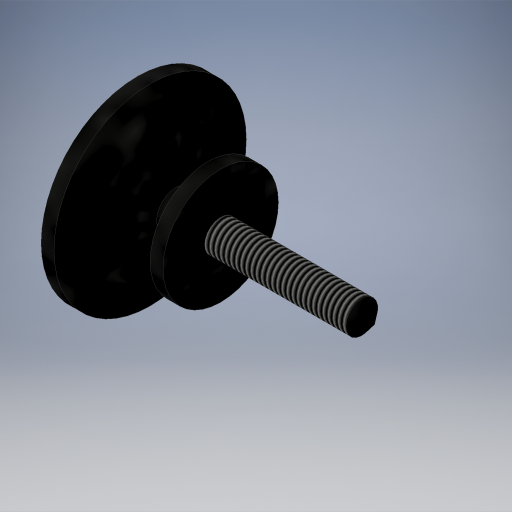
# Autodesk Inventor part: BT002_trajan20_22
Saved by Autodesk Inventor 2023 (Build 270158000, 158)
## iProperties
Company: HTBLA Kaindorf
RuleStatus: InUse
Created: 2022-11-02
Part Number: BT002_trajan20_22
Project: Zeichenmaschine_neu
Material: Kunststoff, undurchsichtig Schwarz
Description: Fuß
Document SubType Name: Modeling
Designer: trajan20
Density: 0.952 g/cm^3
Appearance: Glatt - Schwarz
Mass: 3.50123 g
Surface Area: 26.4974 cm^2
Volume: 3.67776 cm^3
AfterDocNew0: iProperties-Editor_aufrufen
Author: jan
Keywords: 2022
Autodesk Inventor part; units mm, degrees
ref_plane "YZ Plane" through (0, 0, 0) normal (1, 0, 0) x (0, 1, 0)
ref_plane "XZ Plane" through (0, 0, 0) normal (0, 1, 0) x (-1, 0, 0)
ref_plane "XY Plane" through (0, 0, 0) normal (0, 0, 1) x (1, 0, 0)
sketch "Skizze3" plane through (0, 0, 0) normal (0, 0, 1) x (1, 0, 0)
  line L0 (0, 0) -> (15, 0)
  line L1 (15, 0) -> (15, 2)
  line L2 (15, 2) -> (3, 6)
  line L3 (3, 6) -> (3, 11)
  line L4 (3, 11) -> (9, 11)
  line L5 (9, 11) -> (9, 13)
  line L6 (9, 13) -> (2.5, 13)
  line L7 (2.5, 13) -> (2.5, 35)
  line L8 (2.5, 35) -> (0, 37)
  line L9 (0, -1.3947) -> (0, 46.3421)
  dimension "d4" = 18
  dimension "d5" = 6
  dimension "d6" = 2
  dimension "d7" = 5
  dimension "d8" = 2
  dimension "d9" = 6
  dimension "d11" = 5
  dimension "d12" = 30
  dimension "d13" = 35
  dimension "d14" = 2
  constraints: 20 end point, 2 horizontal, 2 parallel, 2 perpendicular, 2 point on line, 2 vertical
  measures "d4" diameter of L5 L9
  measures "d5" distance from line of L0 L2.end
  measures "d6" distance from line of L1.end L0
  measures "d7" distance of L3.end L2.end
  measures "d8" distance between parallel lines of L6 L4
  measures "d9" diameter of L3 L9
  measures "d11" diameter of L7 L9
  measures "d12" diameter of L1 L9
  measures "d13" distance from line of L7.end L0
  measures "d14" vertical distance of L8.end L7.end
revolve "Umdrehung1" add sketch "Skizze3" angle 360 about axis through (0, -1.3947, 0) along (0, 1, 0)
thread "Gewinde1" size "M5x0.8" class "6g" standard "ISO Metric profile" full length
